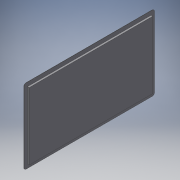
# Autodesk Inventor part: screen
Saved by Autodesk Inventor 2019 (Build 230136000, 136)
## iProperties
Created: 2019-06-25
Part Number: screen
Material: Generic
Document SubType Name: Modeling
Designer: Daniel
Density: 1 g/cm^3
Appearance: Default
Author: Daniel
Autodesk Inventor part; units mm, degrees
ref_plane "YZ Plane" through (0, 0, 0) normal (1, 0, 0) x (0, 1, 0)
ref_plane "XZ Plane" through (0, 0, 0) normal (0, 1, 0) x (-1, 0, 0)
ref_plane "XY Plane" through (0, 0, 0) normal (0, 0, 1) x (1, 0, 0)
sketch "Sketch1" plane through (0, 0, 0) normal (1, 0, 0) x (0, 1, 0)
  line L0 (0, 0) -> (110.744, 0)
  line L1 (110.744, 0) -> (110.744, -193.6242)
  line L2 (110.744, -193.6242) -> (0, -193.6242)
  line L3 (0, -193.6242) -> (0, 0)
  dimension "d0" = 193.6242
  dimension "d1" = 110.744
  constraints: 8 end point, 2 parallel, 1 horizontal, 1 perpendicular
  measures "d0" distance of L0.end L1.end
  measures "d1" distance of L0.start L0.end
extrude "Extrusion1" add sketch "Sketch1" along normal blind 6.1468
fillet "Fillet1" radius 3.175 4 edges at (3.0734, 110.744, 0) (3.0734, 0, 0) (3.0734, 110.744, -193.6242) (3.0734, 0, -193.6242)
sketch "Sketch3" plane through (6.1468, 0, 0) normal (1, 0, 0) x (0, 0, -1)
  arc A0 (3.175, 110.744) -> (0, 107.569) centre (3.175, 107.569) ccw construction
  arc A1 (190.4492, 0) -> (193.6242, 3.175) centre (190.4492, 3.175) ccw construction
  line L0 (3.175, 107.569) -> (190.4492, 3.175) construction
  arc A2 (193.6242, 107.569) -> (190.4492, 110.744) centre (190.4492, 107.569) ccw construction
  arc A3 (0, 3.175) -> (3.175, 0) centre (3.175, 3.175) ccw construction
  line L1 (190.4492, 107.569) -> (3.175, 3.175) construction
  line L2 (5.1644, 5.6494) -> (188.4598, 5.6494)
  line L3 (188.4598, 5.6494) -> (188.4598, 105.0946)
  line L4 (188.4598, 105.0946) -> (5.1644, 105.0946)
  line L5 (5.1644, 105.0946) -> (5.1644, 5.6494)
  line L6 (5.1644, 5.6494) -> (188.4598, 105.0946) construction
  line L7 (188.4598, 5.6494) -> (5.1644, 105.0946) construction
  arc A4 (190.4492, 0) -> (193.6242, 3.175) centre (190.4492, 3.175) ccw projected
  line L8 (193.6242, 3.175) -> (193.6242, 107.569) projected
  arc A5 (193.6242, 107.569) -> (190.4492, 110.744) centre (190.4492, 107.569) ccw projected
  line L9 (190.4492, 110.744) -> (3.175, 110.744) projected
  arc A6 (3.175, 110.744) -> (0, 107.569) centre (3.175, 107.569) ccw projected
  line L10 (0, 107.569) -> (0, 3.175) projected
  arc A7 (0, 3.175) -> (3.175, 0) centre (3.175, 3.175) ccw projected
  line L11 (3.175, 0) -> (190.4492, 0) projected
  point P0 (0, 0)
  point P1 (96.8121, 55.372)
  constraints: 16 end point, 3 midpoint, 2 parallel, 1 horizontal, 1 perpendicular
extrude "Extrusion3" cut sketch "Sketch3" against normal blind 2.54
move faces "Move1" translate (3.175, 0, 0) faces at (0, 36.9147, -65.5997)
body "Solid1"
